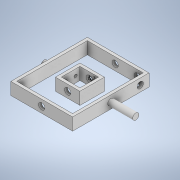
# Autodesk Inventor part: Frame
Saved by Autodesk Inventor 2022 (Build 260153000, 153)
## iProperties
Created: 2023-02-01
Part Number: Frame
Material: Generic
Document SubType Name: Modeling
Designer: Deven Joshi
Density: 1 g/cm^3
Appearance: Default
Author: Deven Joshi
Autodesk Inventor part; units mm, degrees
ref_plane "YZ Plane" through (0, 0, 0) normal (1, 0, 0) x (0, 1, 0)
ref_plane "XZ Plane" through (0, 0, 0) normal (0, 1, 0) x (-1, 0, 0)
ref_plane "XY Plane" through (0, 0, 0) normal (0, 0, 1) x (1, 0, 0)
sketch "Sketch1" plane through (0, 0, 0) normal (0, 1, 0) x (-1, 0, 0)
  line L0 (-63, 78) -> (63, 78)
  line L1 (63, 78) -> (63, -78)
  line L2 (63, -78) -> (-63, -78)
  line L3 (-63, -78) -> (-63, 78)
  line L4 (-63, 78) -> (63, -78) construction
  line L5 (63, 78) -> (-63, -78) construction
  line L6 (-57, 72) -> (57, 72)
  line L7 (57, 72) -> (57, -72)
  line L8 (57, -72) -> (-57, -72)
  line L9 (-57, -72) -> (-57, 72)
  line L10 (-57, 72) -> (57, -72) construction
  line L11 (57, 72) -> (-57, -72) construction
  point P0 (0, 0)
  dimension "d0" = 126
  dimension "d1" = 156
  dimension "d2" = 114
  dimension "d3" = 144
  dimension "d49" = 156
  constraints: 24 end point, 4 midpoint, 4 parallel, 2 horizontal, 2 perpendicular
  measures "d0" distance of L1.end L2.end
  measures "d1" distance of L0.end L1.end
  measures "d2" distance of L7.end L8.end
  measures "d3" distance of L6.end L7.end
  measures "d49" distance of L2.end L0.start
extrude "Extrusion1" add sketch "Sketch1" along normal mid plane 25
sketch "Sketch2" plane through (0, 12.5, 0) normal (0, 1, 0) x (1, 0, 0)
  line L0 (-25, -25) -> (25, -25)
  line L1 (25, -25) -> (25, 25)
  line L2 (25, 25) -> (-25, 25)
  line L3 (-25, 25) -> (-25, -25)
  line L4 (-25, -25) -> (25, 25) construction
  line L5 (25, -25) -> (-25, 25) construction
  line L6 (-19, 19) -> (19, 19)
  line L7 (19, 19) -> (19, -19)
  line L8 (19, -19) -> (-19, -19)
  line L9 (-19, -19) -> (-19, 19)
  point P0 (0, 0)
  dimension "d6" = 50
  dimension "d7" = 50
  dimension "d8" = 6
  constraints: 20 end point, 4 parallel, 2 midpoint, 2 perpendicular, 1 horizontal, 3 other
  measures "d6" distance of L2.end L1.end
  measures "d7" distance of L1.end L0.end
  measures "d8" distance between parallel lines of L2 L6
extrude "Extrusion2" add sketch "Sketch2" against normal blind 25
sketch "Sketch3" plane through (25, 12.5, -25) normal (0, 0, -1) x (-1, 0, 0)
  circle A0 centre (25, -12.5) radius 6.35
  dimension "d11" = 12.7
  constraints: 1 centre point, 1 coincident
  measures "d11" diameter of A0
sketch "Sketch6" plane through (63, -12.5, -78) normal (1, 0, 0) x (0, 0, -1)
  circle A0 centre (-78, 12.5) radius 6.35
  dimension "d22" = 12.7
  constraints: 1 centre point, 1 coincident
  measures "d22" diameter of A0
extrude "Extrusion6" add sketch "Sketch6" along normal blind 51
sketch "Sketch7" plane through (-63, -12.5, 78) normal (-1, 0, 0) x (0, 0, 1)
  circle A0 centre (-78, 12.5) radius 6.35
  dimension "d25" = 12.7
  constraints: 1 centre point, 1 coincident
  measures "d25" diameter of A0
extrude "Extrusion7" add sketch "Sketch7" along normal blind 10
sketch "Sketch8" plane through (63, 12.5, -78) normal (0, 0, -1) x (-1, 0, 0)
  point P0 (63, -12.5)
  point P1 (18, -12.5)
  point P2 (63, -12.5)
  constraints: 1 coincident
hole "Hole1" at (45, 0, -78) direction (0, 0, 1) diameter 12.7 depth 6
sketch "Sketch9" plane through (63, -12.5, -78) normal (1, 0, 0) x (0, 0, -1)
  point P0 (-78, 12.5)
  point P1 (-18, 12.5)
  point P2 (-78, 12.5)
  point P3 (-78, 12.5)
  constraints: 2 coincident
hole "Hole2" at (63, 0, -60) direction (-1, 0, 0) diameter 12.7 depth 6
sketch "Sketch10" plane through (63, 12.5, -78) normal (0, 0, -1) x (-1, 0, 0)
  point P0 (63, -12.5)
  point P1 (63, -12.5)
  constraints: 1 coincident
hole "Hole3" at (0, 0, -78) direction (0, 0, 1) diameter 12.7 end through all
sketch "Sketch11" plane through (-25, 12.5, -25) normal (-1, 0, 0) x (0, 0, 1)
  point P0 (25, -12.5)
  point P1 (15, -12.5)
  point P2 (35, -12.5)
hole "Hole4" at (-25, 0, 10) direction (1, 0, 0) diameter 6.4 depth 6
sketch "Sketch12" plane through (-25, 12.5, -25) normal (-1, 0, 0) x (0, 0, 1)
  point P0 (25, -12.5)
  point P1 (15, -12.5)
hole "Hole5" at (-25, 0, -10) direction (1, 0, 0) diameter 6.4 depth 6
body "Solid1"
